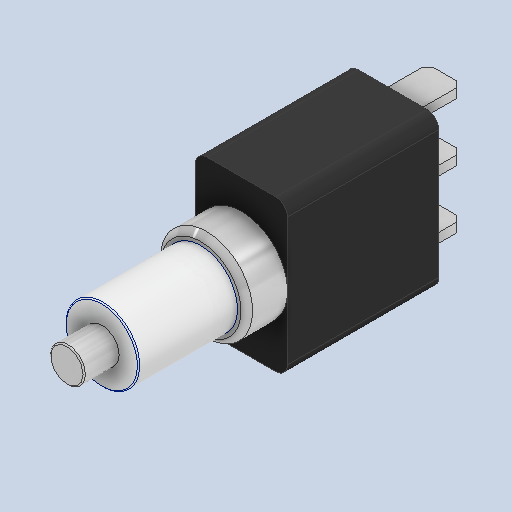
# Autodesk Inventor part: MB2011SD3G01-CA
Saved by Autodesk Inventor 2024.2 (Build 282272000, 272)
## iProperties
Created: 2020-06-24
Part Number: MB2011SD3G01-CA
Material: Generic
Document SubType Name: Modeling
Designer: CASE-SMALL2
Density: 1 g/cm^3
Appearance: Default
Author: CASE-SMALL2
Autodesk Inventor part; units mm, degrees
ref_plane "YZ Plane" through (0, 0, 0) normal (1, 0, 0) x (0, 1, 0)
ref_plane "XZ Plane" through (0, 0, 0) normal (0, 1, 0) x (-1, 0, 0)
ref_plane "XY Plane" through (0, 0, 0) normal (0, 0, 1) x (1, 0, 0)
sketch "Sketch1" plane through (0, 0, 0) normal (0, 0, 1) x (1, 0, 0)
  line L0 (-3.95, -6.5) -> (3.95, -6.5)
  line L1 (3.95, -6.5) -> (3.95, 6.5)
  line L2 (3.95, 6.5) -> (-3.95, 6.5)
  line L3 (-3.95, 6.5) -> (-3.95, -6.5)
  line L4 (-3.95, -6.5) -> (3.95, 6.5) construction
  line L5 (3.95, -6.5) -> (-3.95, 6.5) construction
  point P0 (0, 0)
  dimension "d0" = 13
  dimension "d1" = 7.9
  constraints: 12 end point, 2 midpoint, 2 parallel, 1 horizontal, 1 perpendicular
  measures "d0" distance of L0.end L1.end
  measures "d1" distance of L1.end L2.end
sketch "Sketch1 outline for Extrusion1" plane through (0, 0, 0) normal (0, 0, 1) x (1, 0, 0)
  line L0 (-3.95, -6.5) -> (3.95, -6.5)
  line L1 (-3.95, 6.5) -> (-3.95, -6.5)
  line L2 (3.95, 6.5) -> (-3.95, 6.5)
  line L3 (3.95, -6.5) -> (3.95, 6.5)
extrude "Extrusion1" add sketch "Sketch1 outline for Extrusion1" along normal blind 13
sketch "Sketch2" plane through (0, 0, 0) normal (0, 0, -1) x (-1, 0, 0)
  line L0 (0, -9.1) -> (0, 9.1) projected
  line L1 (-1.5, -5.4) -> (1.5, -5.4)
  line L2 (1.5, -5.4) -> (1.5, -4.6)
  line L3 (1.5, -4.6) -> (-1.5, -4.6)
  line L4 (-1.5, -4.6) -> (-1.5, -5.4)
  line L5 (-1.5, -5.4) -> (1.5, -4.6) construction
  line L6 (1.5, -5.4) -> (-1.5, -4.6) construction
  line L7 (-1.5, -0.4) -> (1.5, -0.4)
  line L8 (1.5, -0.4) -> (1.5, 0.4)
  line L9 (1.5, 0.4) -> (-1.5, 0.4)
  line L10 (-1.5, 0.4) -> (-1.5, -0.4)
  line L11 (-1.5, -0.4) -> (1.5, 0.4) construction
  line L12 (1.5, -0.4) -> (-1.5, 0.4) construction
  line L13 (-1.5, 4.6) -> (1.5, 4.6)
  line L14 (1.5, 4.6) -> (1.5, 5.4)
  line L15 (1.5, 5.4) -> (-1.5, 5.4)
  line L16 (-1.5, 5.4) -> (-1.5, 4.6)
  line L17 (-1.5, 4.6) -> (1.5, 5.4) construction
  line L18 (1.5, 4.6) -> (-1.5, 5.4) construction
  line L19 (-3.95, 6.5) -> (3.95, 6.5) projected
  line L20 (3.95, -6.5) -> (-3.95, -6.5) projected
  point P0 (0, 0)
  point P1 (0, -5)
  point P2 (0, 5)
  dimension "d4" = 1.5
  dimension "d5" = 1.5
  dimension "d6" = 0.8
  dimension "d7" = 0.8
  dimension "d8" = 0.8
  dimension "d9" = 3
  constraints: 36 end point, 6 midpoint, 6 parallel, 4 point on line, 3 horizontal, 3 perpendicular
  measures "d4" distance from line of L19 point (0, 5)
  measures "d5" distance from line of L20 point (0, -5)
  measures "d6" distance of L1.end L2.end
  measures "d7" distance of L7.end L8.end
  measures "d8" distance of L13.end L14.end
  measures "d9" distance of L14.end L15.end
sketch "Sketch2 outline for Extrusion2" plane through (0, 0, 0) normal (0, 0, -1) x (-1, 0, 0)
  line L0 (-1.5, -4.6) -> (-1.5, -5.4)
  line L1 (1.5, -4.6) -> (-1.5, -4.6)
  line L2 (1.5, -5.4) -> (1.5, -4.6)
  line L3 (-1.5, -5.4) -> (1.5, -5.4)
  line L4 (-1.5, 0.4) -> (-1.5, -0.4)
  line L5 (1.5, 0.4) -> (-1.5, 0.4)
  line L6 (1.5, -0.4) -> (1.5, 0.4)
  line L7 (-1.5, -0.4) -> (1.5, -0.4)
  line L8 (-1.5, 5.4) -> (-1.5, 4.6)
  line L9 (1.5, 5.4) -> (-1.5, 5.4)
  line L10 (1.5, 4.6) -> (1.5, 5.4)
  line L11 (-1.5, 4.6) -> (1.5, 4.6)
extrude "Extrusion2" add sketch "Sketch2 outline for Extrusion2" along normal blind 4.5 separate body
sketch "Sketch3" plane through (0, 0, 13) normal (0, 0, 1) x (1, 0, 0)
  circle A0 centre (0, 0) radius 3.95
  line L0 (-3.95, 6.5) -> (-3.95, -6.5) projected
  constraints: 1 centre point, 1 coincident, 1 tangent
sketch "Sketch3 outline for Extrusion3" plane through (0, 0, 13) normal (0, 0, 1) x (1, 0, 0)
  circle A0 centre (0, 0) radius 3.95
extrude "Extrusion3" add sketch "Sketch3 outline for Extrusion3" along normal blind 3.5 separate body
sketch "Sketch4" plane through (0, 0, 16.5) normal (0, 0, 1) x (1, 0, 0)
  circle A0 centre (0, 0) radius 3.15
  dimension "d15" = 6.3
  constraints: 1 centre point, 1 coincident
  measures "d15" diameter of A0
sketch "Sketch4 outline for Extrusion4" plane through (0, 0, 16.5) normal (0, 0, 1) x (1, 0, 0)
  circle A0 centre (0, 0) radius 3.15
extrude "Extrusion4" add sketch "Sketch4 outline for Extrusion4" along normal blind 8.5 separate body
sketch "Sketch5" plane through (0, 0, 25) normal (0, 0, 1) x (1, 0, 0)
  circle A0 centre (0, 0) radius 1.5
  dimension "d18" = 3
  constraints: 1 centre point, 1 coincident
  measures "d18" diameter of A0
sketch "Sketch5 outline for Extrusion5" plane through (0, 0, 25) normal (0, 0, 1) x (1, 0, 0)
  circle A0 centre (0, 0) radius 1.5
extrude "Extrusion5" add sketch "Sketch5 outline for Extrusion5" along normal blind 3 separate body
chamfer "Chamfer1" distance 0.5 angle 45 1 edges at (-3.95, 0, 16.5)
fillet "Fillet1" radius 1 4 edges at (3.95, 6.5, 6.5) (-3.95, 6.5, 6.5) (-3.95, -6.5, 6.5) (3.95, -6.5, 6.5)
chamfer "Chamfer2" distance 0.5 angle 45 6 edges at (-1.5, -5, -4.5) (-1.5, 0, -4.5) (-1.5, 5, -4.5) (1.5, 5, -4.5) (1.5, 0, -4.5) (1.5, -5, -4.5)
fillet "Fillet2" radius 0.1 1 edges at (-1.5, 0, 28)
fillet "Fillet3" radius 0.1 1 edges at (-3.15, 0, 25)
equation "\"d5\" = d4"
equation "\"d7\" = d6"
equation "\"d8\" = d7"
body "Solid1"
body "Solid2"
body "Solid3"
body "Solid4"
body "Solid5"
